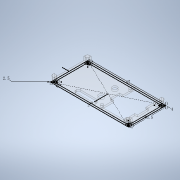
# Autodesk Inventor part: 盖
Saved by Autodesk Inventor 2022 (Build 260153000, 153)
## iProperties
Created: 2022-08-05
Part Number: 盖
Material: 聚碳酸酯，透明
Document SubType Name: Modeling
Designer: Shane
Density: 1.2 g/cm^3
Appearance: 聚碳酸酯 - 透明
Author: Shane
Autodesk Inventor part; units mm, degrees
ref_plane "YZ Plane" through (0, 0, 0) normal (1, 0, 0) x (0, 1, 0)
ref_plane "XZ Plane" through (0, 0, 0) normal (0, 1, 0) x (-1, 0, 0)
ref_plane "XY Plane" through (0, 0, 0) normal (0, 0, 1) x (1, 0, 0)
sketch "草图3" plane through (0, 0, 0) normal (0, 1, 0) x (-1, 0, 0)
  line L0 (40, 20.25) -> (-40, 20.25)
  line L1 (-42.5, 17.75) -> (-42.5, -17.75)
  line L2 (-40, -20.25) -> (40, -20.25)
  line L3 (42.5, -17.75) -> (42.5, 17.75)
  line L4 (42.5, 20.25) -> (-42.5, -20.25) construction
  line L5 (-42.5, 20.25) -> (42.5, -20.25) construction
  arc A0 (42.5, 17.75) -> (40, 20.25) centre (40, 17.75) ccw
  arc A1 (-40, 20.25) -> (-42.5, 17.75) centre (-40, 17.75) ccw
  arc A2 (-42.5, -17.75) -> (-40, -20.25) centre (-40, -17.75) ccw
  arc A3 (40, -20.25) -> (42.5, -17.75) centre (40, -17.75) ccw
  circle A4 centre (40.5, 18.25) radius 1
  line L6 (42.5, 0) -> (50.0267, 0)
  circle A5 centre (40.5, -18.25) radius 1
  line L7 (0, 0) -> (0, 15.1914)
  circle A6 centre (-40.5, 18.25) radius 1
  circle A7 centre (-40.5, -18.25) radius 1
  line L8 (42.5, 20.25) -> (38.5, 20.25)
  line L9 (38.5, 20.25) -> (38.5, 16.25)
  line L10 (38.5, 16.25) -> (42.5, 16.25)
  line L11 (42.5, 16.25) -> (42.5, 20.25)
  line L12 (42.5, 20.25) -> (38.5, 16.25) construction
  line L13 (38.5, 20.25) -> (42.5, 16.25) construction
  line L14 (42.5, -16.25) -> (38.5, -16.25)
  line L15 (38.5, -16.25) -> (38.5, -20.25)
  line L16 (38.5, -20.25) -> (42.5, -20.25)
  line L17 (42.5, -20.25) -> (42.5, -16.25)
  line L18 (42.5, -16.25) -> (38.5, -20.25) construction
  line L19 (38.5, -16.25) -> (42.5, -20.25) construction
  line L20 (-38.5, 20.25) -> (-42.5, 20.25)
  line L21 (-42.5, 20.25) -> (-42.5, 16.25)
  line L22 (-42.5, 16.25) -> (-38.5, 16.25)
  line L23 (-38.5, 16.25) -> (-38.5, 20.25)
  line L24 (-38.5, 20.25) -> (-42.5, 16.25) construction
  line L25 (-42.5, 20.25) -> (-38.5, 16.25) construction
  line L26 (-38.5, -16.25) -> (-42.5, -16.25)
  line L27 (-42.5, -16.25) -> (-42.5, -20.25)
  line L28 (-42.5, -20.25) -> (-38.5, -20.25)
  line L29 (-38.5, -20.25) -> (-38.5, -16.25)
  line L30 (-38.5, -16.25) -> (-42.5, -20.25) construction
  line L31 (-42.5, -16.25) -> (-38.5, -20.25) construction
  line L32 (-36.5, 18.25) -> (36.5, 18.25)
  arc A8 (40.5, 17.75) -> (40, 18.25) centre (40, 17.75) ccw
  line L33 (40.5, 14.25) -> (40.5, -14.25)
  arc A9 (40, -18.25) -> (40.5, -17.75) centre (40, -17.75) ccw
  line L34 (36.5, -18.25) -> (-36.5, -18.25)
  arc A10 (-40.5, -17.75) -> (-40, -18.25) centre (-40, -17.75) ccw
  line L35 (-40.5, -14.25) -> (-40.5, 14.25)
  arc A11 (-40, 18.25) -> (-40.5, 17.75) centre (-40, 17.75) ccw
  arc A12 (-40.5, -14.25) -> (-36.5, -18.25) centre (-36.5, -14.25) ccw
  arc A13 (-36.5, 18.25) -> (-40.5, 14.25) centre (-36.5, 14.25) ccw
  arc A14 (40.5, 14.25) -> (36.5, 18.25) centre (36.5, 14.25) ccw
  arc A15 (36.5, -18.25) -> (40.5, -14.25) centre (36.5, -14.25) ccw
  point P0 (-38.5, -17.7141)
  point P1 (-39.9641, -16.25)
  point P2 (-39.9641, 16.25)
  point P3 (-38.5, 17.7141)
  point P4 (39.9641, -16.25)
  point P5 (38.5, -17.7141)
  point P6 (38.5, 17.7141)
  point P7 (39.9641, 16.25)
  dimension "d11" = 85
  dimension "d12" = 40.5
  dimension "d13" = 2.5
  dimension "d14" = 2
  dimension "d15" = 2
  dimension "d16" = 2
  dimension "d72" = 4
  dimension "d73" = 4
  dimension "d74" = 4
  dimension "d75" = 4
  dimension "d76" = 4
  dimension "d77" = 4
  dimension "d78" = 4
  dimension "d79" = 4
  dimension "d80" = 2
  dimension "d81" = 4
  constraints: 72 end point, 24 point on circle, 16 centre point, 16 point on line, 16 tangent, 12 parallel, 11 midpoint, 6 equal radius, 6 horizontal, 6 perpendicular, 3 symmetric about line, 1 vertical, 10 other
  measures "d11" distance of L5.end L4.end
  measures "d12" distance of L4.end L5.start
  measures "d13" radius of A0
  measures "d14" diameter of A4
  measures "d15" distance from line of L0 A4.centre
  measures "d16" distance from line of L3 A4.centre
  measures "d72" distance of L10.end L9.end
  measures "d73" distance of L9.end L8.end
  measures "d74" distance of L16.end L15.end
  measures "d75" distance of L15.end L14.end
  measures "d76" distance of L22.end L21.end
  measures "d77" distance of L21.end L20.end
  measures "d78" distance of L28.end L4.end
  measures "d79" distance of L4.end L26.end
  measures "d80" distance between parallel lines of L0 L32
  measures "d81" radius of A12
extrude "拉伸3" add sketch "草图3" along normal blind 2 contours A0 L3 L10 A14 L9 L0 | L9 A14 L32 A13 L23 L0 | L23 A13 L22 L1 A1 L0 | A14 L10 L9 | L9 L10 A14 L33 A15 L14 L15 L34 A12 L29 L26 L35 A13 L22 L23 L32 | L3 L14 A15 L33 A14 L10 | L23 L22 A13 | A13 L35 A12 L26 L1 L22 | L3 A3 L2 L15 A15 L14 | A15 L15 L14 | L26 A12 L29 L2 A2 L1 | L15 L2 L29 A12 L34 A15 | L26 L29 A12 | A4 | A5 | A6 | A7
extrude "拉伸4" add sketch "草图3" along normal blind 6 contours A0 L3 L10 A14 L9 L0 | L8 L11 A0 | L23 A13 L22 L1 A1 L0 | A1 L21 L20 | L3 A3 L2 L15 A15 L14 | L17 L16 A3 | L26 A12 L29 L2 A2 L1 | A2 L28 L27 | A4 | A5 | A6 | A7
sketch "草图4" plane through (0, 0, 0) normal (0, -1, 0) x (1, 0, 0)
  line L0 (40.5, -20.1774) -> (40.5, 20.25)
  line L1 (-38.5, 20.25) -> (38.5, 20.25) projected
  line L2 (42.5, 17.75) -> (42.5, -17.75) projected
  line L3 (38.5, -20.25) -> (-38.5, -20.25) projected
  line L4 (6.5, -20.25) -> (6.5, 20.25)
  circle A0 centre (38, -15.5) radius 1.5
  line L5 (40.5, -18) -> (25.2781, -18)
  line L6 (25.2781, -18) -> (6.5, -18)
  line L7 (6.5, 18) -> (40.5, 18)
  line L8 (23.5, 18) -> (23.5, -18)
  circle A1 centre (9, -15.5) radius 1.5
  circle A2 centre (9, 15.5) radius 1.5
  circle A3 centre (38, 15.5) radius 1.5
  line L9 (11.4, -18) -> (11.4, 18)
  line L10 (35.4, -18) -> (35.4, 18)
  line L11 (35.4, -6) -> (38.1, -6)
  line L12 (38.1, -6) -> (38.1, 6)
  line L13 (38.1, 6) -> (35.4, 6)
  line L14 (6.5, -5) -> (9.5, -5)
  line L15 (9.5, -5) -> (9.5, 5)
  line L16 (9.5, 5) -> (6.5, 5)
  line L17 (7.5, -5) -> (11.5, -5)
  line L18 (11.5, -5) -> (11.5, 5)
  line L19 (11.5, 5) -> (7.5, 5)
  line L20 (7.5, 5) -> (7.5, -5)
  line L21 (7.5, -5) -> (11.5, 5) construction
  line L22 (11.5, -5) -> (7.5, 5) construction
  point P0 (0, 0)
  point P1 (-40, 20.25)
  point P2 (40, 20.25)
  point P3 (40, -20.25)
  point P4 (-40, -20.25)
  point P5 (9.5, 0)
  point P6 (7.5, 5)
  point P7 (7.5, -5)
  dimension "d21" = 2
  dimension "d22" = 34
  dimension "d23" = 3
  dimension "d24" = 2.5
  dimension "d25" = 18
  dimension "d26" = 2.5
  dimension "d27" = 18
  dimension "d28" = 3
  dimension "d29" = 3
  dimension "d30" = 3
  dimension "d31" = 2.5
  dimension "d32" = 2.5
  dimension "d33" = 2.5
  dimension "d34" = 2.5
  dimension "d35" = 2.5
  dimension "d36" = 2.5
  dimension "d37" = 2.4
  dimension "d38" = 24
  dimension "d39" = 2.7
  dimension "d40" = 6
  dimension "d41" = 12
  dimension "d42" = 3
  dimension "d43" = 5
  dimension "d44" = 10
  dimension "d45" = 4
  dimension "d46" = 10
  constraints: 40 end point, 16 point on line, 9 perpendicular, 4 centre point, 4 midpoint, 4 vertical, 3 horizontal, 2 parallel
  measures "d21" distance between parallel lines of L2 L0
  measures "d22" distance between parallel lines of L4 L0
  measures "d23" diameter of A0
  measures "d24" distance from line of L0 A0.centre
  measures "d25" distance from line of point (0, 0) L5
  measures "d26" distance from line of L5 A0.centre
  measures "d27" distance from line of point (0, 0) L7
  measures "d28" diameter of A1
  measures "d29" diameter of A2
  measures "d30" diameter of A3
  measures "d31" distance from line of L6 A1.centre
  measures "d32" distance from line of L4 A1.centre
  measures "d33" distance from line of L4 A2.centre
  measures "d34" distance from line of L7 A2.centre
  measures "d35" distance from line of L0 A3.centre
  measures "d36" distance from line of L7 A3.centre
  measures "d37" distance from line of L9 A1.centre
  measures "d38" distance between parallel lines of L10 L9
  measures "d39" distance of L11.start L11.end
  measures "d40" distance from line of point (0, 0) L11
  measures "d41" distance of L11.end L12.end
  measures "d42" distance of L14.start L14.end
  measures "d43" distance from line of point (0, 0) L14
  measures "d44" distance of L14.end L15.end
  measures "d45" distance of L19.end L18.end
  measures "d46" distance of L18.end L17.end
extrude "拉伸5" cut sketch "草图4" against normal blind 2 contours L5 L6 L8 L7 L10 | L10 L13 L12 L11 | L8 L6 L9 L17 L18 L19 L7 | L19 L18 L17 L9 | L9 L17 L15 L19 | L15 L14 L20 L16 | A0 | A1 | A2 | A3
fillet "圆角6" radius 2.5 4 edges at (-42.5, 3, -20.25) (-42.5, 3, 20.25) (42.5, 3, 20.25) (42.5, 3, -20.25)
sketch "草图6" plane through (0, 0, 0) normal (0, -1, 0) x (1, 0, 0)
  line L0 (-40, 20.25) -> (40, 20.25) projected
  line L1 (0, 20.25) -> (-19, 20.25)
  line L2 (-19, 20.25) -> (-19, 13.25)
  line L3 (-19, 13.25) -> (0, 13.25)
  line L4 (0, 13.25) -> (0, 20.25)
  line L5 (0, 13.25) -> (3, 13.25)
  line L6 (3, 13.25) -> (3, 20.25)
  line L7 (3, 20.25) -> (0, 20.25)
  line L8 (0, 20.25) -> (0, 13.25)
  line L9 (3, 20.25) -> (3, 18.25)
  line L10 (3, 18.25) -> (-19, 18.25)
  point P0 (0, 0)
  dimension "d83" = 19
  dimension "d84" = 7
  dimension "d85" = 3
  dimension "d86" = 7
  dimension "d87" = 2
  constraints: 20 end point, 4 parallel, 3 perpendicular, 2 horizontal, 2 point on line, 1 midpoint
  measures "d83" distance of L3.end L2.end
  measures "d84" distance of L2.end L1.end
  measures "d85" distance of L7.end L6.end
  measures "d86" distance of L6.end L5.end
  measures "d87" distance of L6.end L9.end
extrude "拉伸7" cut sketch "草图6" against normal blind 2 contours L10 L4 L3 L2 | L10 L6 L5 L4
fillet "圆角7" radius 2 4 edges at (3, 1, 13.25) (3, 1, 18.25) (-19, 1, 13.25) (-19, 1, 18.25)
sketch "草图7" plane through (0, 0, 0) normal (0, -1, 0) x (1, 0, 0)
  circle A0 centre (0, 0) radius 7.5
  circle A1 centre (0, -7.5) radius 2.6
  circle A2 centre (0, 7.5) radius 2.6
  dimension "d91" = 5.2
  dimension "d92" = 5.2
  constraints: 3 centre point, 2 point on circle, 1 coincident
  measures "d91" diameter of A1
  measures "d92" diameter of A2
extrude "拉伸8" cut sketch "草图7" against normal blind 2 contours A2 A0 | A0 A2 | A1 A0 | A0 A1
